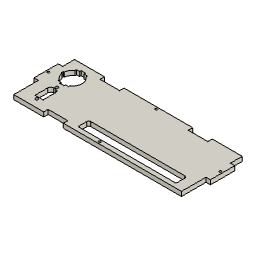
Back Plate (Autodesk Fusion 360 design; units mm, degrees)
Autodesk Fusion 360 part; units mm, degrees
note: some values were not read from the file. Chosen so that the rebuilt part matches the saved one: that a step has no effect. Set by a fixed rule: which sketch regions a step uses.
sketch "Sketch1" plane through (0, 0, 0) normal (0, 0, 1) x (1, 0, 0)
  line L0 (90, -31) -> (-90, -31)
  line L1 (-90, -31) -> (-90, 31)
  line L2 (-90, 31) -> (90, 31)
  line L3 (90, 31) -> (90, -31)
  line L4 (90, -31) -> (-90, 31) construction
  line L5 (-90, -31) -> (90, 31) construction
  line L6 (-90, 26.5) -> (90, 26.5)
  line L7 (90, -26.5) -> (-90, -26.5)
  line L8 (-85.5, 31) -> (-85.5, -31)
  line L9 (85.5, -31) -> (85.5, 31)
  line L10 (-90, 31) -> (-55, 31)
  line L11 (-55, 31) -> (-55, 26.5)
  line L12 (-55, 26.5) -> (-90, 26.5)
  line L13 (-90, 26.5) -> (-90, 31)
  line L14 (-55, 26.5) -> (-35, 26.5)
  line L15 (-35, 26.5) -> (-35, 31)
  line L16 (-35, 31) -> (-55, 31)
  line L17 (-55, 31) -> (-55, 26.5)
  line L18 (90, 31) -> (55, 31)
  line L19 (55, 31) -> (55, 26.5)
  line L20 (55, 26.5) -> (90, 26.5)
  line L21 (90, 26.5) -> (90, 31)
  line L22 (55, 26.5) -> (35, 26.5)
  line L23 (35, 26.5) -> (35, 31)
  line L24 (35, 31) -> (55, 31)
  line L25 (55, 31) -> (55, 26.5)
  line L26 (-90, -31) -> (-55, -31)
  line L27 (-55, -31) -> (-55, -26.5)
  line L28 (-55, -26.5) -> (-90, -26.5)
  line L29 (-90, -26.5) -> (-90, -31)
  line L30 (-55, -26.5) -> (-35, -26.5)
  line L31 (-35, -26.5) -> (-35, -31)
  line L32 (-35, -31) -> (-55, -31)
  line L33 (-55, -31) -> (-55, -26.5)
  line L34 (55, -26.5) -> (90, -26.5)
  line L35 (90, -26.5) -> (90, -31)
  line L36 (90, -31) -> (85.5, -31)
  line L37 (85.5, -31) -> (85.5, -6)
  line L38 (85.5, -6) -> (90, -6)
  line L39 (90, -6) -> (90, -31)
  line L40 (85.5, -6) -> (90, -6)
  line L41 (90, -6) -> (90, 19)
  line L42 (90, 19) -> (85.5, 19)
  line L43 (85.5, 19) -> (85.5, -6)
  line L44 (-90, -31) -> (-85.5, -31)
  line L45 (-85.5, -31) -> (-85.5, -6)
  line L46 (-85.5, -6) -> (-90, -6)
  line L47 (-90, -6) -> (-90, -31)
  line L48 (-90, -6) -> (-85.5, -6)
  line L49 (-85.5, -6) -> (-85.5, 19)
  line L50 (-85.5, 19) -> (-90, 19)
  line L51 (-90, 19) -> (-90, -6)
  line L52 (87.75, 35) -> (87.75, -35) construction
  line L53 (-87.75, 42) -> (-87.75, -36) construction
  line L54 (-97, 28.75) -> (95, 28.75) construction
  line L55 (95, -28.75) -> (-97, -28.75) construction
  circle A0 centre (87.75, 6.5) radius 1.15
  circle A1 centre (-87.75, 6.5) radius 1.15
  circle A2 centre (0, 28.75) radius 1.15
  circle A3 centre (0, -28.75) radius 1.15
  circle A4 centre (-70, 13.5) radius 9.75
  line L56 (-64.5, 23) -> (-75.5, 23)
  line L57 (-75.5, 23) -> (-75.5, 4)
  line L58 (-75.5, 4) -> (-64.5, 4)
  line L59 (-64.5, 4) -> (-64.5, 23)
  line L60 (-64.5, 23) -> (-75.5, 4) construction
  line L61 (-75.5, 23) -> (-64.5, 4) construction
  line L62 (-67.75, 2.5) -> (-72.25, 2.5)
  line L63 (-72.25, 2.5) -> (-72.25, 24.5)
  line L64 (-72.25, 24.5) -> (-67.75, 24.5)
  line L65 (-67.75, 24.5) -> (-67.75, 2.5)
  line L66 (-67.75, 2.5) -> (-72.25, 24.5) construction
  line L67 (-72.25, 2.5) -> (-67.75, 24.5) construction
  line L68 (-80.75, 12.4) -> (-59.25, 12.4)
  line L69 (-59.25, 12.4) -> (-59.25, 14.6)
  line L70 (-59.25, 14.6) -> (-80.75, 14.6)
  line L71 (-80.75, 14.6) -> (-80.75, 12.4)
  line L72 (-80.75, 12.4) -> (-59.25, 14.6) construction
  line L73 (-59.25, 12.4) -> (-80.75, 14.6) construction
  line L74 (-70, 35) -> (-70, -35) construction
  line L75 (-65.9, -20.75) -> (-74.1, -20.75)
  line L76 (-74.1, -20.75) -> (-74.1, -7.75)
  line L77 (-71.1, -4.75) -> (-68.9, -4.75)
  line L78 (-65.9, -7.75) -> (-65.9, -20.75)
  line L79 (-65.9, -20.75) -> (-74.1, -4.75) construction
  line L80 (-74.1, -20.75) -> (-65.9, -4.75) construction
  circle A5 centre (-70, -2.5) radius 1.4
  circle A6 centre (-70, -23) radius 1.4
  circle A7 centre (-70, 13.5) radius 11.5 construction
  arc A8 (-71.1, -4.75) -> (-74.1, -7.75) centre (-71.1, -7.75) ccw
  arc A9 (-65.9, -7.75) -> (-68.9, -4.75) centre (-68.9, -7.75) ccw
  line L81 (-24.5, -26.5) -> (75.5, -26.5)
  line L82 (75.5, -26.5) -> (75.5, -15.5)
  line L83 (75.5, -15.5) -> (-24.5, -15.5)
  line L84 (-24.5, -15.5) -> (-24.5, -26.5)
  point P0 (-70, 13.5)
  point P1 (-70, 13.5)
  point P2 (-70, 13.5)
  point P3 (-70, -12.75)
  point P4 (0, 5)
  point P5 (0, 5)
  point P6 (0, 20.0443)
  point P7 (-41, 5)
  dimension "d1" = 180
  dimension "d2" = 62
  dimension "d3" = 4.5
  dimension "d4" = 4.5
  dimension "d5" = 4.5
  dimension "d6" = 4.5
  dimension "d7" = 35
  dimension "d8" = 20
  dimension "d9" = 35
  dimension "d10" = 20
  dimension "d11" = 35
  dimension "d12" = 20
  dimension "d15" = 25
  dimension "d16" = 25
  dimension "d17" = 25
  dimension "d18" = 25
  dimension "d21" = 2.25
  dimension "d22" = 2.25
  dimension "d23" = 2.25
  dimension "d24" = 2.25
  dimension "d25" = 2.3
  dimension "d26" = 2.3
  dimension "d27" = 2.3
  dimension "d28" = 2.3
  dimension "d29" = 35
  dimension "d30" = 35
  dimension "d31" = 37.5
  dimension "d32" = 37.5
  dimension "d33" = 19.5
  dimension "d34" = 11
  dimension "d35" = 19
  dimension "d36" = 4.5
  dimension "d37" = 22
  dimension "d38" = 21.5
  dimension "d39" = 2.2
  dimension "d40" = 20
  dimension "d41" = 8.2
  dimension "d42" = 16
  dimension "d43" = 2.8
  dimension "d44" = 2.8
  dimension "d45" = 10.25
  dimension "d46" = 10.25
  dimension "d47" = 3.5
  dimension "d48" = 23
  dimension "d58" = 3
  dimension "d59" = 3
  dimension "d69" = 100
  dimension "d70" = 11
  dimension "d71" = 10
  dimension "d123" = 40
  constraint horizontal L0
  constraint perpendicular L0 L1
  constraint parallel L0 L2
  constraint parallel L1 L3
  constraint coincident L4 origin
  constraint coincident L5 origin
  constraint perpendicular L1 L6
  constraint perpendicular L1 L7
  constraint perpendicular L7 L8
  constraint parallel L8 L9
  constraint horizontal L10
  constraint vertical L11
  constraint horizontal L12
  constraint vertical L13
  constraint horizontal L14
  constraint vertical L15
  constraint horizontal L16
  constraint vertical L17
  constraint horizontal L18
  constraint vertical L19
  constraint horizontal L20
  constraint vertical L21
  constraint horizontal L22
  constraint vertical L23
  constraint horizontal L24
  constraint vertical L25
  constraint horizontal L26
  constraint vertical L27
  constraint horizontal L28
  constraint vertical L29
  constraint horizontal L30
  constraint vertical L31
  constraint horizontal L32
  constraint vertical L33
  constraint horizontal L34
  constraint vertical L35
  constraint horizontal L36
  constraint vertical L37
  constraint horizontal L38
  constraint vertical L39
  constraint horizontal L40
  constraint vertical L41
  constraint horizontal L42
  constraint vertical L43
  constraint horizontal L44
  constraint vertical L45
  constraint horizontal L46
  constraint vertical L47
  constraint horizontal L48
  constraint vertical L49
  constraint horizontal L50
  constraint vertical L51
  constraint coincident L8.start L10
  constraint parallel L47 L53
  constraint horizontal L54
  constraint parallel L0 L55
  constraint coincident L52 A0.centre
  constraint coincident L53 A1.centre
  constraint coincident L54 A2.centre
  constraint coincident L55 A3.centre
  constraint horizontal L56
  constraint perpendicular L56 L57
  constraint parallel L56 L58
  constraint parallel L57 L59
  constraint coincident L60 P2
  constraint coincident L61 P2
  constraint coincident P2 P1
  constraint horizontal L62
  constraint perpendicular L62 L63
  constraint parallel L62 L64
  constraint parallel L63 L65
  constraint coincident L66 P2
  constraint coincident L67 P2
  constraint horizontal L68
  constraint perpendicular L68 L69
  constraint parallel L68 L70
  constraint parallel L69 L71
  constraint coincident L72 P2
  constraint coincident L73 P2
  constraint perpendicular L0 L74
  constraint coincident P2 L74
  constraint horizontal L75
  constraint perpendicular L75 L76
  constraint parallel L75 L77
  constraint parallel L76 L78
  constraint coincident L79 P3
  constraint coincident L80 P3
  constraint coincident L74 P3
  constraint coincident L74 A5.centre
  constraint coincident L74 A6.centre
  constraint coincident L79.end L77
  constraint coincident L79.end L76
  constraint tangent L77 A8
  constraint tangent L76 A8
  constraint coincident L80.end L77
  constraint coincident L80.end L78
  constraint tangent L77 A9
  constraint tangent L78 A9
  constraint horizontal L81
  constraint vertical L82
  constraint horizontal L83
  constraint vertical L84
  constraint coincident L7 L81.start
  constraint collinear L2 L24
  constraint collinear L2 L16
  constraint collinear L0 L32
  constraint coincident L2 L9.end
  constraint coincident P5 P4
  constraint vertical origin P5
  measures "d1" distance of L1.end L2.end
  measures "d2" distance of L0.end L1.end
  measures "d3" distance of L3 L9
  measures "d4" distance of L1 L8
  measures "d5" distance of L2 L6
  measures "d6" distance of L0 L7
  measures "d7" distance of L1.end L10.end
  measures "d8" distance of L11.end L14.end
  measures "d9" distance of L2.end L18.end
  measures "d10" distance of L19.end L22.end
  measures "d11" distance of L0.end L26.end
  measures "d12" distance of L27.end L30.end
  measures "d15" distance of L0.start L38.end
  measures "d16" distance of L37.end L42.end
  measures "d17" distance of L0.end L46.end
  measures "d18" distance of L46.end L50.end
  measures "d21" distance of L1 L53
  measures "d22" distance of L3 L52
  measures "d23" distance of L0 L55
  measures "d24" distance of L2 L54
  measures "d25" diameter of A0
  measures "d26" diameter of A1
  measures "d27" diameter of A2
  measures "d28" diameter of A3
  measures "d29" distance of L15 A2.centre
  measures "d30" distance of L31 A3.centre
  measures "d31" distance of L0 A0.centre
  measures "d32" distance of L44 A1.centre
  measures "d33" diameter of A4
  measures "d34" distance of L57.end L58.end
  measures "d35" distance of L56.end L57.end
  measures "d36" distance of L63.end L64.end
  measures "d37" distance of L62.end L63.end
  measures "d38" distance of L69.end L70.end
  measures "d39" distance of L68.end L69.end
  measures "d40" distance of L1 L74
  measures "d41" distance of L79.end L80.end
  measures "d42" distance of L75.end L79.end
  measures "d43" diameter of A5
  measures "d44" diameter of A6
  measures "d45" distance of P3 A6.centre
  measures "d46" distance of P3 A5.centre
  measures "d47" distance of L7 A6.centre
  measures "d48" diameter of A7
  measures "d58" radius of A8
  measures "d59" radius of A9
  measures "d69" distance of L81.start L81.end
  measures "d70" distance of L81.start L83.end
  measures "d71" distance of L37 L82
  measures "d123" distance of L28 P2
extrude "Extrude1" add sketch "Sketch1" along normal blind 4.5 contours L0 L7 L9 L31 L34 L37 L81 | L6 L7 L8 L9 L12 L14 L20 L22 L28 L30 L34 L37 L43 L45 L49 L82 L83 L84 | L3 L9 L38 L40 L41 L42 L43 | L0 L7 L8 L26 L27 L28 L33 L45 | L2 L6 L9 L18 L19 L20 L25 | L1 L8 L46 L48 L49 L50 L51 | L2 L6 L15 L23 | L2 L6 L8 L10 L11 L12 L17 | A4 L68 L69 L70 | A4 L56 L65 | A4 L58 L65 | A4 L56 L63 | A4 L58 L63
move_face "OffsetFaces1" offset -0.1 2 faces at (87, -6, 3) (-87, -6, 3)
move_face "OffsetFaces2" offset -0.1 2 faces at (-87, 19, 1.5) (88.5, 19, 1.5)
fillet "Fillet1" radius 2 2 edges at (-24.5, -15.5, 2.25) (75.5, -15.5, 2.25)
fillet "Fillet2" radius 1 2 edges at (75.5, -26.5, 2.25) (-24.5, -26.5, 2.25)
fillet "Fillet3" radius 0.2 2 edges at (-74.1, -20.75, 2.25) (-65.9, -20.75, 2.25)
fillet "Fillet4" [no effect]
sketch "Sketch3" plane through (0, 0, 4.5) normal (0, 0, 1) x (-1, 0, 0)
  line L0 (75.5, -23) -> (72.25, -23)
  line L1 (72.25, -23) -> (72.25, -24.5)
  line L2 (72.25, -24.5) -> (67.75, -24.5)
  line L3 (67.75, -24.5) -> (67.75, -23)
  line L4 (67.75, -23) -> (64.5, -23)
  line L5 (64.5, -23) -> (64.5, -21.5506)
  arc A0 (64.5, -5.4494) -> (64.5, -21.5506) centre (70, -13.5) ccw
  line L6 (64.5, -5.4494) -> (64.5, -4)
  line L7 (64.5, -4) -> (67.75, -4)
  line L8 (67.75, -4) -> (67.75, -2.5)
  line L9 (67.75, -2.5) -> (72.25, -2.5)
  line L10 (72.25, -2.5) -> (72.25, -4)
  line L11 (72.25, -4) -> (75.5, -4)
  line L12 (75.5, -4) -> (75.5, -5.4494)
  arc A1 (79.6877, -12.4) -> (75.5, -5.4494) centre (70, -13.5) ccw
  line L13 (79.6877, -12.4) -> (80.75, -12.4)
  line L14 (80.75, -12.4) -> (80.75, -14.6)
  line L15 (80.75, -14.6) -> (79.6877, -14.6)
  arc A2 (75.5, -21.5506) -> (79.6877, -14.6) centre (70, -13.5) ccw
  line L16 (75.5, -21.5506) -> (75.5, -23)
  line L17 (65.9, 7.75) -> (65.9, 20.55)
  arc A3 (66.1, 20.75) -> (65.9, 20.55) centre (66.1, 20.55) ccw
  line L18 (66.1, 20.75) -> (73.9, 20.75)
  arc A4 (74.1, 20.55) -> (73.9, 20.75) centre (73.9, 20.55) ccw
  line L19 (74.1, 20.55) -> (74.1, 7.75)
  arc A5 (71.1, 4.75) -> (74.1, 7.75) centre (71.1, 7.75) ccw
  line L20 (71.1, 4.75) -> (68.9, 4.75)
  arc A6 (65.9, 7.75) -> (68.9, 4.75) centre (68.9, 7.75) ccw
  circle A7 centre (0, -28.75) radius 1.15
  circle A8 centre (87.75, -6.5) radius 1.15
  circle A9 centre (0, 28.75) radius 1.15
  circle A10 centre (70, 2.5) radius 1.4
  line L21 (24.5, 25.5) -> (24.5, 17.5)
  arc A11 (22.5, 15.5) -> (24.5, 17.5) centre (22.5, 17.5) ccw
  line L22 (22.5, 15.5) -> (-73.5, 15.5)
  arc A12 (-75.5, 17.5) -> (-73.5, 15.5) centre (-73.5, 17.5) ccw
  line L23 (-75.5, 17.5) -> (-75.5, 25.5)
  arc A13 (-74.5, 26.5) -> (-75.5, 25.5) centre (-74.5, 25.5) ccw
  line L24 (-74.5, 26.5) -> (23.5, 26.5)
  arc A14 (24.5, 25.5) -> (23.5, 26.5) centre (23.5, 25.5) ccw
  circle A15 centre (-87.75, -6.5) radius 1.15
  circle A16 centre (70, 23) radius 1.4
  line L25 (85.5, -31) -> (85.5, -18.9)
  line L26 (85.5, -18.9) -> (90, -18.9)
  line L27 (90, -18.9) -> (90, 5.9)
  line L28 (90, 5.9) -> (85.5, 5.9)
  line L29 (85.5, 5.9) -> (85.5, 31)
  line L30 (85.5, 31) -> (55, 31)
  line L31 (55, 31) -> (55, 26.5)
  line L32 (55, 26.5) -> (35, 26.5)
  line L33 (35, 26.5) -> (35, 31)
  line L34 (35, 31) -> (-85.5, 31)
  line L35 (-85.5, 31) -> (-85.5, 5.9)
  line L36 (-85.5, 5.9) -> (-90, 5.9)
  line L37 (-90, 5.9) -> (-90, -18.9)
  line L38 (-90, -18.9) -> (-85.5, -18.9)
  line L39 (-85.5, -18.9) -> (-85.5, -31)
  line L40 (-85.5, -31) -> (-55, -31)
  line L41 (-55, -31) -> (-55, -26.5)
  line L42 (-55, -26.5) -> (-35, -26.5)
  line L43 (-35, -26.5) -> (-35, -31)
  line L44 (-35, -31) -> (35, -31)
  line L45 (35, -31) -> (35, -26.5)
  line L46 (35, -26.5) -> (55, -26.5)
  line L47 (55, -26.5) -> (55, -31)
  line L48 (55, -31) -> (85.5, -31)
  line L49 (81.2036, 5.2559) -> (82.162, 5.2559)
  line L50 (82.162, 5.2559) -> (82.162, 1.644)
  spline S0 degree 2 poles (82.162, 1.644) (82.6872, 2.1351) (83.4001, 2.3705) knots 0 0 0 1 1 1
  line L51 (83.4001, 2.3705) -> (83.4001, 1.5008)
  spline S1 degree 2 poles (83.4001, 1.5008) (83.0249, 1.378) (82.5849, 1.0369) knots 0 0 0 1 1 1
  spline S2 degree 2 poles (82.5849, 1.0369) (82.145, 0.6924) (81.9812, 0.2354) knots 0 0 0 1 1 1
  line L52 (81.9812, 0.2354) -> (81.2036, 0.2354)
  line L53 (81.2036, 0.2354) -> (81.2036, 5.2559)
  line L54 (76.5345, 4.3657) -> (76.5345, 5.2559)
  line L55 (76.5345, 5.2559) -> (79.8939, 5.2559)
  spline S3 degree 2 poles (79.8939, 5.2559) (79.8394, 4.7511) (79.5665, 4.3009) knots 0 0 0 1 1 1
  spline S4 degree 2 poles (79.5665, 4.3009) (79.2937, 3.8473) (78.4887, 3.1003) knots 0 0 0 1 1 1
  spline S5 degree 2 poles (78.4887, 3.1003) (77.8407, 2.4967) (77.6941, 2.2818) knots 0 0 0 1 1 1
  spline S6 degree 2 poles (77.6941, 2.2818) (77.4963, 1.9851) (77.4963, 1.6952) knots 0 0 0 1 1 1
  spline S7 degree 2 poles (77.4963, 1.6952) (77.4963, 1.3746) (77.6702, 1.204) knots 0 0 0 1 1 1
  spline S8 degree 2 poles (77.6702, 1.204) (77.8407, 1.0301) (78.1443, 1.0301) knots 0 0 0 1 1 1
  spline S9 degree 2 poles (78.1443, 1.0301) (78.4444, 1.0301) (78.6218, 1.2109) knots 0 0 0 1 1 1
  spline S10 degree 2 poles (78.6218, 1.2109) (78.7991, 1.3916) (78.8264, 1.8111) knots 0 0 0 1 1 1
  line L56 (78.8264, 1.8111) -> (79.7814, 1.7156)
  spline S11 degree 2 poles (79.7814, 1.7156) (79.6961, 0.9244) (79.2459, 0.5799) knots 0 0 0 1 1 1
  spline S12 degree 2 poles (79.2459, 0.5799) (78.7957, 0.2354) (78.1204, 0.2354) knots 0 0 0 1 1 1
  spline S13 degree 2 poles (78.1204, 0.2354) (77.3803, 0.2354) (76.9574, 0.6345) knots 0 0 0 1 1 1
  spline S14 degree 2 poles (76.9574, 0.6345) (76.5345, 1.0335) (76.5345, 1.6269) knots 0 0 0 1 1 1
  spline S15 degree 2 poles (76.5345, 1.6269) (76.5345, 1.9646) (76.6572, 2.2716) knots 0 0 0 1 1 1
  spline S16 degree 2 poles (76.6572, 2.2716) (76.7766, 2.5751) (77.0392, 2.9094) knots 0 0 0 1 1 1
  spline S17 degree 2 poles (77.0392, 2.9094) (77.2132, 3.131) (77.6668, 3.5471) knots 0 0 0 1 1 1
  spline S18 degree 2 poles (77.6668, 3.5471) (78.1204, 3.9632) (78.2432, 4.0997) knots 0 0 0 1 1 1
  spline S19 degree 2 poles (78.2432, 4.0997) (78.3626, 4.2361) (78.4376, 4.3657) knots 0 0 0 1 1 1
  line L57 (78.4376, 4.3657) -> (76.5345, 4.3657)
  line L58 (75.7909, 3.9223) -> (75.7909, 2.9639)
  line L59 (75.7909, 2.9639) -> (73.9083, 2.9639)
  line L60 (73.9083, 2.9639) -> (73.9083, 3.9223)
  line L61 (73.9083, 3.9223) -> (75.7909, 3.9223)
  line L62 (70.3237, 4.3657) -> (70.3237, 5.2559)
  line L63 (70.3237, 5.2559) -> (73.6832, 5.2559)
  spline S20 degree 2 poles (73.6832, 5.2559) (73.6286, 4.7511) (73.3557, 4.3009) knots 0 0 0 1 1 1
  spline S21 degree 2 poles (73.3557, 4.3009) (73.0829, 3.8473) (72.278, 3.1003) knots 0 0 0 1 1 1
  spline S22 degree 2 poles (72.278, 3.1003) (71.6299, 2.4967) (71.4833, 2.2818) knots 0 0 0 1 1 1
  spline S23 degree 2 poles (71.4833, 2.2818) (71.2855, 1.9851) (71.2855, 1.6952) knots 0 0 0 1 1 1
  spline S24 degree 2 poles (71.2855, 1.6952) (71.2855, 1.3746) (71.4594, 1.204) knots 0 0 0 1 1 1
  spline S25 degree 2 poles (71.4594, 1.204) (71.6299, 1.0301) (71.9335, 1.0301) knots 0 0 0 1 1 1
  spline S26 degree 2 poles (71.9335, 1.0301) (72.2336, 1.0301) (72.411, 1.2109) knots 0 0 0 1 1 1
  spline S27 degree 2 poles (72.411, 1.2109) (72.5883, 1.3916) (72.6156, 1.8111) knots 0 0 0 1 1 1
  line L64 (72.6156, 1.8111) -> (73.5706, 1.7156)
  spline S28 degree 2 poles (73.5706, 1.7156) (73.4853, 0.9244) (73.0351, 0.5799) knots 0 0 0 1 1 1
  spline S29 degree 2 poles (73.0351, 0.5799) (72.5849, 0.2354) (71.9096, 0.2354) knots 0 0 0 1 1 1
  spline S30 degree 2 poles (71.9096, 0.2354) (71.1695, 0.2354) (70.7466, 0.6345) knots 0 0 0 1 1 1
  spline S31 degree 2 poles (70.7466, 0.6345) (70.3237, 1.0335) (70.3237, 1.6269) knots 0 0 0 1 1 1
  spline S32 degree 2 poles (70.3237, 1.6269) (70.3237, 1.9646) (70.4465, 2.2716) knots 0 0 0 1 1 1
  spline S33 degree 2 poles (70.4465, 2.2716) (70.5658, 2.5751) (70.8284, 2.9094) knots 0 0 0 1 1 1
  spline S34 degree 2 poles (70.8284, 2.9094) (71.0024, 3.131) (71.456, 3.5471) knots 0 0 0 1 1 1
  spline S35 degree 2 poles (71.456, 3.5471) (71.9096, 3.9632) (72.0324, 4.0997) knots 0 0 0 1 1 1
  spline S36 degree 2 poles (72.0324, 4.0997) (72.1518, 4.2361) (72.2268, 4.3657) knots 0 0 0 1 1 1
  line L65 (72.2268, 4.3657) -> (70.3237, 4.3657)
  line L66 (67.7964, 5.2559) -> (67.7964, 4.2497)
  line L67 (67.7964, 4.2497) -> (69.8428, 4.2497)
  line L68 (69.8428, 4.2497) -> (69.8428, 3.4107)
  line L69 (69.8428, 3.4107) -> (67.6736, 0.2354)
  line L70 (67.6736, 0.2354) -> (66.8687, 0.2354)
  line L71 (66.8687, 0.2354) -> (66.8687, 3.4073)
  line L72 (66.8687, 3.4073) -> (66.248, 3.4073)
  line L73 (66.248, 3.4073) -> (66.248, 4.2497)
  line L74 (66.248, 4.2497) -> (66.8687, 4.2497)
  line L75 (66.8687, 4.2497) -> (66.8687, 5.2559)
  line L76 (66.8687, 5.2559) -> (67.7964, 5.2559)
  line L77 (67.7964, 3.4073) -> (67.7964, 1.6986)
  line L78 (67.7964, 1.6986) -> (68.9458, 3.4073)
  line L79 (68.9458, 3.4073) -> (67.7964, 3.4073)
  line L80 (64.3039, 5.2559) -> (66.0911, 0.2559)
  line L81 (66.0911, 0.2559) -> (64.9963, 0.2559)
  line L82 (64.9963, 0.2559) -> (63.7309, 3.9564)
  line L83 (63.7309, 3.9564) -> (62.5065, 0.2559)
  line L84 (62.5065, 0.2559) -> (61.4355, 0.2559)
  line L85 (61.4355, 0.2559) -> (63.2261, 5.2559)
  line L86 (63.2261, 5.2559) -> (64.3039, 5.2559)
  line L87 (57.6054, 5.2559) -> (58.4956, 5.2559)
  line L88 (58.4956, 5.2559) -> (58.4956, 4.7238)
  spline S37 degree 2 poles (58.4956, 4.7238) (58.7173, 5.0342) (59.0208, 5.1877) knots 0 0 0 1 1 1
  spline S38 degree 2 poles (59.0208, 5.1877) (59.3209, 5.3377) (59.6279, 5.3377) knots 0 0 0 1 1 1
  spline S39 degree 2 poles (59.6279, 5.3377) (60.252, 5.3377) (60.6988, 4.8364) knots 0 0 0 1 1 1
  spline S40 degree 2 poles (60.6988, 4.8364) (61.1422, 4.3316) (61.1422, 3.4312) knots 0 0 0 1 1 1
  spline S41 degree 2 poles (61.1422, 3.4312) (61.1422, 2.5103) (60.7091, 2.0328) knots 0 0 0 1 1 1
  spline S42 degree 2 poles (60.7091, 2.0328) (60.2759, 1.5519) (59.6143, 1.5519) knots 0 0 0 1 1 1
  spline S43 degree 2 poles (59.6143, 1.5519) (59.0072, 1.5519) (58.5638, 2.0567) knots 0 0 0 1 1 1
  line L89 (58.5638, 2.0567) -> (58.5638, 0.2559)
  line L90 (58.5638, 0.2559) -> (57.6054, 0.2559)
  line L91 (57.6054, 0.2559) -> (57.6054, 5.2559)
  spline S44 degree 2 poles (60.1634, 3.3664) (60.1634, 3.9462) (60.0031, 4.2054) knots 0 0 0 1 1 1
  spline S45 degree 2 poles (60.0031, 4.2054) (59.7711, 4.5806) (59.355, 4.5806) knots 0 0 0 1 1 1
  spline S46 degree 2 poles (59.355, 4.5806) (59.0242, 4.5806) (58.7923, 4.3009) knots 0 0 0 1 1 1
  spline S47 degree 2 poles (58.7923, 4.3009) (58.5604, 4.0178) (58.5604, 3.4585) knots 0 0 0 1 1 1
  spline S48 degree 2 poles (58.5604, 3.4585) (58.5604, 2.8343) (58.7855, 2.5615) knots 0 0 0 1 1 1
  spline S49 degree 2 poles (58.7855, 2.5615) (59.0106, 2.2852) (59.3619, 2.2852) knots 0 0 0 1 1 1
  spline S50 degree 2 poles (59.3619, 2.2852) (59.7029, 2.2852) (59.9349, 2.5581) knots 0 0 0 1 1 1
  spline S51 degree 2 poles (59.9349, 2.5581) (60.1634, 2.8275) (60.1634, 3.3664) knots 0 0 0 1 1 1
  line L92 (53.5024, 2.7047) -> (54.4471, 2.8752)
  spline S52 degree 2 poles (54.4471, 2.8752) (54.4949, 2.5922) (54.6654, 2.4489) knots 0 0 0 1 1 1
  spline S53 degree 2 poles (54.6654, 2.4489) (54.8325, 2.3057) (55.102, 2.3057) knots 0 0 0 1 1 1
  spline S54 degree 2 poles (55.102, 2.3057) (55.4601, 2.3057) (55.675, 2.5546) knots 0 0 0 1 1 1
  spline S55 degree 2 poles (55.675, 2.5546) (55.8864, 2.8002) (55.8864, 3.38) knots 0 0 0 1 1 1
  spline S56 degree 2 poles (55.8864, 3.38) (55.8864, 4.0246) (55.6716, 4.2907) knots 0 0 0 1 1 1
  spline S57 degree 2 poles (55.6716, 4.2907) (55.4533, 4.5567) (55.0883, 4.5567) knots 0 0 0 1 1 1
  spline S58 degree 2 poles (55.0883, 4.5567) (54.8155, 4.5567) (54.6415, 4.4032) knots 0 0 0 1 1 1
  spline S59 degree 2 poles (54.6415, 4.4032) (54.4676, 4.2463) (54.396, 3.8677) knots 0 0 0 1 1 1
  line L93 (54.396, 3.8677) -> (53.4546, 4.028)
  spline S60 degree 2 poles (53.4546, 4.028) (53.6013, 4.6761) (54.0174, 5.0069) knots 0 0 0 1 1 1
  spline S61 degree 2 poles (54.0174, 5.0069) (54.4335, 5.3377) (55.1327, 5.3377) knots 0 0 0 1 1 1
  spline S62 degree 2 poles (55.1327, 5.3377) (55.9274, 5.3377) (56.4014, 4.8364) knots 0 0 0 1 1 1
  spline S63 degree 2 poles (56.4014, 4.8364) (56.8721, 4.335) (56.8721, 3.4482) knots 0 0 0 1 1 1
  spline S64 degree 2 poles (56.8721, 3.4482) (56.8721, 2.5512) (56.398, 2.0533) knots 0 0 0 1 1 1
  spline S65 degree 2 poles (56.398, 2.0533) (55.9239, 1.5519) (55.1156, 1.5519) knots 0 0 0 1 1 1
  spline S66 degree 2 poles (55.1156, 1.5519) (54.454, 1.5519) (54.0651, 1.8384) knots 0 0 0 1 1 1
  spline S67 degree 2 poles (54.0651, 1.8384) (53.6729, 2.1215) (53.5024, 2.7047) knots 0 0 0 1 1 1
emboss "Emboss1" [suppressed]
equation "d45 = ( 20.5 / 2 ) * 1 mm"
equation "d46 = ( 20.5 / 2 ) * 1 mm"
